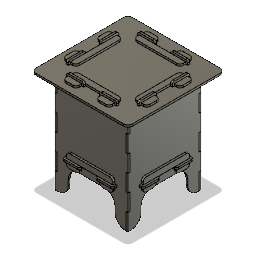
Laterne in 3D parametrisiert (Autodesk Fusion 360 design; units mm, degrees)
Autodesk Fusion 360 part; units mm, degrees
note: some values were not read from the file. Set by a fixed rule: which sketch regions a step uses.
sketch "Skizze1" plane through (0, 0, 0) normal (0, 1, 0) x (1, 0, 0)
  line L0 (52, -52) -> (-52, -52)
  line L1 (-52, -52) -> (-52, 52)
  line L2 (-52, 52) -> (52, 52)
  line L3 (52, 52) -> (52, -52)
  line L4 (52, -52) -> (-52, 52) construction
  line L5 (-52, -52) -> (52, 52) construction
  line L6 (-12, 52) -> (-38, 52)
  line L7 (-38, 52) -> (-38, 58)
  line L8 (-35, 61) -> (-15, 61)
  line L9 (-12, 58) -> (-12, 52)
  line L10 (0, 52) -> (0, -52) construction
  line L11 (-52, 0) -> (52, 0) construction
  line L12 (-35, 55) -> (-15, 55)
  line L13 (-15, 55) -> (-15, 58)
  line L14 (-15, 58) -> (-35, 58)
  line L15 (-35, 58) -> (-35, 55)
  arc A0 (-35, 61) -> (-38, 58) centre (-35, 58) ccw
  arc A1 (-12, 58) -> (-15, 61) centre (-15, 58) ccw
  line L16 (38, 52) -> (38, 58)
  arc A2 (38, 58) -> (35, 61) centre (35, 58) ccw
  line L17 (35, 61) -> (15, 61)
  arc A3 (15, 61) -> (12, 58) centre (15, 58) ccw
  line L18 (12, 58) -> (12, 52)
  line L19 (35, 55) -> (15, 55)
  line L20 (15, 55) -> (15, 58)
  line L21 (15, 58) -> (35, 58)
  line L22 (35, 58) -> (35, 55)
  line L23 (55, 35) -> (55, 15)
  line L24 (55, 15) -> (58, 15)
  line L25 (58, 12) -> (52, 12)
  line L26 (52, 38) -> (58, 38)
  line L27 (61, 35) -> (61, 15)
  arc A4 (61, 35) -> (58, 38) centre (58, 35) ccw
  arc A5 (58, 12) -> (61, 15) centre (58, 15) ccw
  line L28 (58, 35) -> (55, 35)
  line L29 (58, 15) -> (58, 35)
  line L30 (52, -38) -> (58, -38)
  line L31 (61, -35) -> (61, -15)
  line L32 (55, -35) -> (55, -15)
  line L33 (55, -15) -> (58, -15)
  line L34 (58, -15) -> (58, -35)
  arc A6 (61, -15) -> (58, -12) centre (58, -15) ccw
  arc A7 (58, -38) -> (61, -35) centre (58, -35) ccw
  line L35 (58, -35) -> (55, -35)
  line L36 (58, -12) -> (52, -12)
  line L37 (-35, -55) -> (-15, -55)
  line L38 (-35, -61) -> (-15, -61)
  line L39 (-15, -55) -> (-15, -58)
  line L40 (-35, -58) -> (-35, -55)
  arc A8 (-38, -58) -> (-35, -61) centre (-35, -58) ccw
  line L41 (-12, -58) -> (-12, -52)
  line L42 (-38, -52) -> (-38, -58)
  line L43 (35, -61) -> (15, -61)
  line L44 (-15, -58) -> (-35, -58)
  line L45 (12, -58) -> (12, -52)
  line L46 (35, -55) -> (15, -55)
  line L47 (35, -58) -> (35, -55)
  line L48 (15, -55) -> (15, -58)
  arc A9 (-15, -61) -> (-12, -58) centre (-15, -58) ccw
  arc A10 (35, -61) -> (38, -58) centre (35, -58) ccw
  arc A11 (12, -58) -> (15, -61) centre (15, -58) ccw
  line L49 (15, -58) -> (35, -58)
  line L50 (38, -52) -> (38, -58)
  arc A12 (-58, 38) -> (-61, 35) centre (-58, 35) ccw
  line L51 (-55, 15) -> (-58, 15)
  line L52 (-55, -35) -> (-55, -15)
  line L53 (-55, 35) -> (-55, 15)
  line L54 (-58, 35) -> (-55, 35)
  line L55 (-55, -15) -> (-58, -15)
  line L56 (-58, -35) -> (-55, -35)
  line L57 (-58, -15) -> (-58, -35)
  arc A13 (-61, 15) -> (-58, 12) centre (-58, 15) ccw
  line L58 (-58, 12) -> (-52, 12)
  line L59 (-58, 15) -> (-58, 35)
  arc A14 (-61, -35) -> (-58, -38) centre (-58, -35) ccw
  line L60 (-61, -35) -> (-61, -15)
  line L61 (-52, 38) -> (-58, 38)
  line L62 (-58, -12) -> (-52, -12)
  arc A15 (-58, -12) -> (-61, -15) centre (-58, -15) ccw
  line L63 (-61, 35) -> (-61, 15)
  line L64 (-52, -38) -> (-58, -38)
  point P0 (-38, 61)
  point P1 (-12, 61)
  point P2 (61, -38)
  point P3 (61, -12)
  point P4 (12, -61)
  point P5 (38, -61)
  point P6 (-52, -52)
  point P7 (-61, 38)
  point P8 (-52, 0)
  point P9 (-61, 12)
  dimension "d5" = 104
  dimension "d6" = 104
  dimension "d8" = 9
  dimension "d9" = 26
  dimension "d12" = 3
  dimension "d13" = 20
  dimension "d14" = 3
  dimension "d15" = 3
  dimension "d16" = 3
  dimension "d28" = 15
  measures "d5" distance of L1.end L2.end
  measures "d6" distance of P6 L1.end
  measures "d8" distance of L6.start P1
  measures "d9" distance of P0 P1
  measures "d12" distance of L7 L15
  measures "d13" distance of L12.start L12.end
  measures "d14" distance of L6 L12
  measures "d15" distance of L12.end L13.end
  measures "d16" radius of A0
  measures "d28" distance of L10 L13
extrude "Extrusion1" add sketch "Skizze1" along normal blind 3 makes body 1 in component "Boden"
sketch "Skizze2" plane through (-52, 0, 0) normal (-1, 0, 0) x (0, 0, 1)
  line L0 (-12, 0) -> (12, 0) construction
  line L1 (12, 0) -> (12, 3) construction
  line L2 (12, 3) -> (-12, 3)
  line L3 (-12, 3) -> (-12, 0)
  line L4 (-55, 3) -> (55, 3) construction
  line L5 (55, 3) -> (55, 103)
  line L6 (55, 103) -> (-55, 103)
  line L7 (-55, 103) -> (-55, 3)
  line L8 (-55, 3) -> (55, 103) construction
  line L9 (55, 3) -> (-55, 103) construction
  line L10 (-58, 3) -> (-52, 3)
  line L11 (0, 53) -> (0, 3) construction
  line L12 (0, 3) -> (0, 0) construction
  line L13 (-55, 3) -> (55, 3) construction
  line L14 (55, 3) -> (55, 0) construction
  line L15 (-55, 0) -> (-55, 3)
  line L16 (-38, 103) -> (-12, 103)
  line L17 (-12, 103) -> (-12, 109)
  line L18 (-15, 112) -> (-35, 112)
  line L19 (-38, 109) -> (-38, 103)
  line L20 (0, 53) -> (0, 103) construction
  line L21 (-35, 109) -> (-15, 109)
  line L22 (-15, 109) -> (-15, 106)
  line L23 (-15, 106) -> (-35, 106)
  line L24 (-35, 106) -> (-35, 109)
  arc A0 (-35, 112) -> (-38, 109) centre (-35, 109) ccw
  arc A1 (-12, 109) -> (-15, 112) centre (-15, 109) ccw
  line L25 (15, 112) -> (35, 112)
  line L26 (35, 106) -> (35, 109)
  line L27 (38, 109) -> (38, 103)
  line L28 (15, 106) -> (35, 106)
  line L29 (15, 109) -> (15, 106)
  arc A2 (38, 109) -> (35, 112) centre (35, 109) ccw
  line L30 (12, 103) -> (12, 109)
  arc A3 (15, 112) -> (12, 109) centre (15, 109) ccw
  line L31 (35, 109) -> (15, 109)
  line L32 (-35, -26) -> (-35, -34)
  line L33 (-51, -50) -> (-55, -50)
  line L34 (-55, -50) -> (-55, 0)
  line L35 (35, -26) -> (35, -34)
  line L36 (51, -50) -> (55, -50)
  line L37 (55, -50) -> (55, 0)
  line L38 (19, -10) -> (-19, -10)
  arc A4 (-51, -50) -> (-35, -34) centre (-51, -34) ccw
  arc A5 (35, -34) -> (51, -50) centre (51, -34) ccw
  arc A6 (-19, -10) -> (-35, -26) centre (-19, -26) ccw
  arc A7 (35, -26) -> (19, -10) centre (19, -26) ccw
  line L39 (55, 103) -> (52, 103)
  line L40 (52, 103) -> (52, -50)
  line L41 (52, -50) -> (55, -50)
  line L42 (55, -50) -> (55, 103)
  line L43 (-55, 103) -> (-52, 103)
  line L44 (-52, 103) -> (-52, -50)
  line L45 (-52, -50) -> (-55, -50)
  line L46 (-55, -50) -> (-55, 103)
  line L47 (-55, 0) -> (55, 0) construction
  line L48 (55, 77.5) -> (52, 77.5)
  line L49 (55, 52) -> (52, 52)
  line L50 (55, 26.5) -> (52, 26.5)
  line L51 (55, 1) -> (52, 1)
  line L52 (55, -24.5) -> (52, -24.5)
  line L53 (-55, 77.5) -> (-52, 77.5)
  line L54 (-55, 52) -> (-52, 52)
  line L55 (-55, 26.5) -> (-52, 26.5)
  line L56 (-55, 1) -> (-52, 1)
  line L57 (-55, -24.5) -> (-52, -24.5)
  point P0 (0, 53)
  point P1 (55, 0)
  point P2 (-35, -50)
  point P3 (35, -50)
  dimension "d19" = 110
  dimension "d21" = 100
  dimension "d29" = 9
  dimension "d30" = 20
  dimension "d31" = 3
  dimension "d32" = 3
  dimension "d33" = 3
  dimension "d34" = 3
  dimension "d35" = 15
  dimension "d36" = 3
  dimension "d43" = 20
  dimension "d44" = 20
  dimension "d47" = 16
  dimension "d49" = 16
  dimension "d51" = 3
  dimension "d52" = 3
  dimension "d66" = 50
  dimension "d67" = 3
  dimension "d68" = 25.5
  dimension "d71" = -25.5
  dimension "d72" = 0
  dimension "d73" = 40
  dimension "d74" = 3
  measures "d19" distance of L5.end L6.end
  measures "d21" distance of L4.end L5.end
  measures "d29" distance of L16 L18
  measures "d30" distance of L22 L24
  measures "d31" distance of L19 L24
  measures "d32" distance of L17 L22
  measures "d33" distance of L16 L23
  measures "d34" distance of L21 L23
  measures "d35" distance of L20 L22
  measures "d36" radius of A0
  measures "d43" distance of P2 L33.end
  measures "d44" distance of P3 L36.end
  measures "d47" radius of A4
  measures "d49" radius of A6
  measures "d51" distance of L5.end L39.end
  measures "d52" distance of L44 L46
  measures "d66" distance of L36 L47
  measures "d67" distance of L48.start L48.end
  measures "d68" distance of L6 L48
  measures "d73" distance of L36 L38
  measures "d74" distance of L4 L47
extrude "Extrusion1'" add sketch "Skizze2" along normal blind 3 separate body contours L5 L40 L42 L49 L50 | L37 L40 L42 L51 L52 | L6 L16 L32 L33 L35 L36 L38 A4 A5 A6 A7 L40 L44 | L5 L6 L39 L40 L42 L48 | L6 L25 L27 A2 L30 A3 | L6 L16 L17 L18 L19 A0 A1 | L7 L44 L46 L53 L54 | L7 L10 L44 L46 L55 | L33 L34 L44 L45 L46 L57 | L10 L15 L44 L46 L56 makes body 2 in component "Seite"
combine "Kombinieren1" operation cut target body 2 tool bodies 1 keep tools in component "Seite"
other "C-Anordnung2"
sketch "Skizze4" plane through (0, 103, 0) normal (0, 1, 0) x (-1, 0, 0)
  line L0 (55, -52) -> (38, -52)
  line L1 (38, -52) -> (38, -55)
  line L2 (38, -55) -> (55, -55)
  line L3 (55, -55) -> (55, -52)
  line L4 (-66, 73) -> (66, 73)
  line L5 (73, 66) -> (73, -66)
  line L6 (66, -73) -> (-66, -73)
  line L7 (-73, -66) -> (-73, 66)
  line L8 (-73, 73) -> (73, -73) construction
  line L9 (70.898, 70.898) -> (-73, -73) construction
  arc A0 (-73, -66) -> (-66, -73) centre (-66, -66) ccw
  arc A1 (-66, 73) -> (-73, 66) centre (-66, 66) ccw
  arc A2 (73, 66) -> (66, 73) centre (66, 66) ccw
  arc A3 (66, -73) -> (73, -66) centre (66, -66) ccw
  dimension "d79" = 146
  dimension "d80" = 146
  dimension "d83" = 7
  dimension "d86" = 73
  dimension "d87" = 85
  measures "d79" distance of L8.end L9.end
  measures "d80" distance of L8.start L9.end
  measures "d83" radius of A0
  measures "d86" distance of origin L4
extrude "Extrusion1''" add sketch "Skizze4" along normal blind 3 separate body contours L0 L1 L2 L3 | L4 L5 L6 L7 A0 A1 A2 A3 makes body 3 in component "Deckel"
combine "Kombinieren1'" operation cut target body 3 tool bodies 2 keep tools in component "Deckel"
combine "Kombinieren2" operation cut target body 3 tool bodies 2 body 2 seen with x (0, 0, -1) y (0, 1, 0) z (1, 0, 0) at (0, 0, 0) keep tools in component "Deckel"
combine "Kombinieren3" operation cut target body 3 tool bodies 2 body 2 seen with x (-1, 0, 0) y (0, 1, 0) z (0, 0, -1) at (0, 0, 0) keep tools in component "Deckel"
combine "Kombinieren4" operation cut target body 3 tool bodies 2 body 2 seen with x (0, 0, 1) y (0, 1, 0) z (-1, 0, 0) at (0, 0, 0) keep tools in component "Deckel"
sketch "Skizze5" plane through (0, 106, 0) normal (0, 1, 0) x (-1, 0, 0)
  line L0 (-38, -52) -> (-12, -52)
  line L1 (-12, -52) -> (-12, -55)
  line L2 (-12, -55) -> (-38, -55)
  line L3 (-38, -55) -> (-38, -52)
  line L4 (12, -52) -> (38, -52)
  line L5 (38, -52) -> (38, -55)
  line L6 (38, -55) -> (12, -55)
  line L7 (12, -55) -> (12, -52)
  line L8 (-52, 38) -> (-52, 12)
  line L9 (-52, 12) -> (-55, 12)
  line L10 (-55, 12) -> (-55, 38)
  line L11 (-55, 38) -> (-52, 38)
  line L12 (-52, -12) -> (-52, -38)
  line L13 (-52, -38) -> (-55, -38)
  line L14 (-55, -38) -> (-55, -12)
  line L15 (-55, -12) -> (-52, -12)
  line L16 (38, 52) -> (12, 52)
  line L17 (12, 52) -> (12, 55)
  line L18 (12, 55) -> (38, 55)
  line L19 (38, 55) -> (38, 52)
  line L20 (-12, 52) -> (-38, 52)
  line L21 (-38, 52) -> (-38, 55)
  line L22 (-38, 55) -> (-12, 55)
  line L23 (-12, 55) -> (-12, 52)
  line L24 (52, -38) -> (52, -12)
  line L25 (52, -12) -> (55, -12)
  line L26 (55, -12) -> (55, -38)
  line L27 (55, -38) -> (52, -38)
  line L28 (52, 12) -> (52, 38)
  line L29 (52, 38) -> (55, 38)
  line L30 (55, 38) -> (55, 12)
  line L31 (55, 12) -> (52, 12)
  arc A0 (-73, -66) -> (-66, -73) centre (-66, -66) ccw
  line L32 (-66, -73) -> (66, -73)
  arc A1 (66, -73) -> (73, -66) centre (66, -66) ccw
  line L33 (73, -66) -> (73, 66)
  arc A2 (73, 66) -> (66, 73) centre (66, 66) ccw
  line L34 (66, 73) -> (-66, 73)
  arc A3 (-66, 73) -> (-73, 66) centre (-66, 66) ccw
  line L35 (-73, 66) -> (-73, -66)
  line L36 (35, 45) -> (35, 35)
  line L37 (30, 30) -> (-30, 30)
  line L38 (-35, 35) -> (-35, 45)
  line L39 (-30, 50) -> (-20, 50)
  line L40 (-15, 45) -> (-15, 38.5)
  line L41 (-15, 38.5) -> (15, 38.5)
  line L42 (15, 38.5) -> (15, 45)
  line L43 (20, 50) -> (30, 50)
  arc A4 (30, 30) -> (35, 35) centre (30, 35) ccw
  arc A5 (-35, 35) -> (-30, 30) centre (-30, 35) ccw
  arc A6 (-30, 50) -> (-35, 45) centre (-30, 45) ccw
  arc A7 (-15, 45) -> (-20, 50) centre (-20, 45) ccw
  arc A8 (20, 50) -> (15, 45) centre (20, 45) ccw
  arc A9 (35, 45) -> (30, 50) centre (30, 45) ccw
  point P0 (35, 50)
  point P1 (-35, 50)
  point P2 (-15, 50)
  point P3 (15, 50)
  dimension "d88" = 20
  dimension "d89" = 20
  dimension "d90" = 30
  dimension "d92" = 5
  dimension "d94" = 20
  dimension "d95" = 8.5
  measures "d88" distance of P1 P2
  measures "d89" distance of P0 P3
  measures "d90" distance of L40.end L41.end
  measures "d92" radius of A4
  measures "d94" distance of L37 L43
  measures "d95" distance of L37 L41
extrude "Extrusion1'''" add sketch "Skizze5" along normal blind 3 separate body contours L36 L37 L38 L39 L40 L41 L42 L43 A4 A5 A6 A7 A8 A9 makes body 4 in component "Riegel"
other "C-Anordnung3"
other "C-Anordnung4"
sketch "Skizze6" plane through (0, 3, 0) normal (0, 1, 0) x (-1, 0, 0)
  line L0 (15, 55) -> (15, 58)
  line L1 (15, 58) -> (35, 58)
  line L2 (35, 58) -> (35, 55)
  line L3 (35, 55) -> (15, 55)
  line L4 (35, -55) -> (35, -58)
  line L5 (35, -58) -> (15, -58)
  line L6 (15, -58) -> (15, -55)
  line L7 (15, -55) -> (35, -55)
  line L8 (58, 35) -> (58, 15)
  line L9 (58, 15) -> (55, 15)
  line L10 (55, 15) -> (55, 35)
  line L11 (55, 35) -> (58, 35)
  line L12 (-58, 15) -> (-58, 35)
  line L13 (-58, 35) -> (-55, 35)
  line L14 (-55, 35) -> (-55, 15)
  line L15 (-55, 15) -> (-58, 15)
  line L16 (-35, 58) -> (-15, 58)
  line L17 (-15, 58) -> (-15, 55)
  line L18 (-15, 55) -> (-35, 55)
  line L19 (-35, 55) -> (-35, 58)
  line L20 (-58, -35) -> (-58, -15)
  line L21 (-58, -15) -> (-55, -15)
  line L22 (-55, -15) -> (-55, -35)
  line L23 (-55, -35) -> (-58, -35)
  line L24 (55, -15) -> (58, -15)
  line L25 (58, -15) -> (58, -35)
  line L26 (58, -35) -> (55, -35)
  line L27 (55, -35) -> (55, -15)
  line L28 (-15, -58) -> (-35, -58)
  line L29 (-35, -58) -> (-35, -55)
  line L30 (-35, -55) -> (-15, -55)
  line L31 (-15, -55) -> (-15, -58)
  line L32 (38, 52) -> (38, 58)
  arc A0 (38, 58) -> (35, 61) centre (35, 58) ccw
  line L33 (35, 61) -> (15, 61)
  arc A1 (15, 61) -> (12, 58) centre (15, 58) ccw
  line L34 (12, 58) -> (12, 52)
  line L35 (12, 52) -> (-12, 52)
  line L36 (-12, 52) -> (-12, 58)
  arc A2 (-12, 58) -> (-15, 61) centre (-15, 58) ccw
  line L37 (-15, 61) -> (-35, 61)
  arc A3 (-35, 61) -> (-38, 58) centre (-35, 58) ccw
  line L38 (-38, 58) -> (-38, 52)
  line L39 (-38, 52) -> (-52, 52)
  line L40 (-52, 52) -> (-52, 38)
  line L41 (-52, 38) -> (-58, 38)
  arc A4 (-58, 38) -> (-61, 35) centre (-58, 35) ccw
  line L42 (-61, 35) -> (-61, 15)
  arc A5 (-61, 15) -> (-58, 12) centre (-58, 15) ccw
  line L43 (-58, 12) -> (-52, 12)
  line L44 (-52, 12) -> (-52, -12)
  line L45 (-52, -12) -> (-58, -12)
  arc A6 (-58, -12) -> (-61, -15) centre (-58, -15) ccw
  line L46 (-61, -15) -> (-61, -35)
  arc A7 (-61, -35) -> (-58, -38) centre (-58, -35) ccw
  line L47 (-58, -38) -> (-52, -38)
  line L48 (-52, -38) -> (-52, -52)
  line L49 (-52, -52) -> (-38, -52)
  line L50 (-38, -52) -> (-38, -58)
  arc A8 (-38, -58) -> (-35, -61) centre (-35, -58) ccw
  line L51 (-35, -61) -> (-15, -61)
  arc A9 (-15, -61) -> (-12, -58) centre (-15, -58) ccw
  line L52 (-12, -58) -> (-12, -52)
  line L53 (-12, -52) -> (12, -52)
  line L54 (12, -52) -> (12, -58)
  arc A10 (12, -58) -> (15, -61) centre (15, -58) ccw
  line L55 (15, -61) -> (35, -61)
  arc A11 (35, -61) -> (38, -58) centre (35, -58) ccw
  line L56 (38, -58) -> (38, -52)
  line L57 (38, -52) -> (52, -52)
  line L58 (52, -52) -> (52, -38)
  line L59 (52, -38) -> (58, -38)
  arc A12 (58, -38) -> (61, -35) centre (58, -35) ccw
  line L60 (61, -35) -> (61, -15)
  arc A13 (61, -15) -> (58, -12) centre (58, -15) ccw
  line L61 (58, -12) -> (52, -12)
  line L62 (52, -12) -> (52, 12)
  line L63 (52, 12) -> (58, 12)
  arc A14 (58, 12) -> (61, 15) centre (58, 15) ccw
  line L64 (61, 15) -> (61, 35)
  arc A15 (61, 35) -> (58, 38) centre (58, 35) ccw
  line L65 (58, 38) -> (52, 38)
  line L66 (52, 38) -> (52, 52)
  line L67 (52, 52) -> (38, 52)
sketch "Skizze7" plane through (-55, 0, 0) normal (-1, 0, 0) x (0, 0, 1)
  line L0 (12, 0) -> (12, 3)
  line L1 (12, 3) -> (38, 3)
  line L2 (38, 3) -> (38, 0)
  line L3 (38, 0) -> (12, 0)
  line L4 (-38, 0) -> (-38, 3)
  line L5 (-38, 3) -> (-12, 3)
  line L6 (-12, 3) -> (-12, 0)
  line L7 (-12, 0) -> (-38, 0)
  line L8 (-15, 106) -> (-35, 106)
  line L9 (-35, 106) -> (-35, 109)
  line L10 (-35, 109) -> (-15, 109)
  line L11 (-15, 109) -> (-15, 106)
  line L12 (15, 109) -> (35, 109)
  line L13 (35, 109) -> (35, 106)
  line L14 (35, 106) -> (15, 106)
  line L15 (15, 106) -> (15, 109)
  arc A0 (-51, -50) -> (-35, -34) centre (-51, -34) ccw
  line L16 (-35, -34) -> (-35, -26)
  arc A1 (-19, -10) -> (-35, -26) centre (-19, -26) ccw
  line L17 (-19, -10) -> (19, -10)
  arc A2 (35, -26) -> (19, -10) centre (19, -26) ccw
  line L18 (35, -26) -> (35, -34)
  arc A3 (35, -34) -> (51, -50) centre (51, -34) ccw
  line L19 (52, -50) -> (52, -24.5)
  line L20 (52, -24.5) -> (55, -24.5)
  line L21 (55, -24.5) -> (55, 1)
  line L22 (55, 1) -> (52, 1)
  line L23 (52, 1) -> (52, 26.5)
  line L24 (52, 26.5) -> (55, 26.5)
  line L25 (55, 26.5) -> (55, 52)
  line L26 (55, 52) -> (52, 52)
  line L27 (52, 52) -> (52, 77.5)
  line L28 (52, 77.5) -> (55, 77.5)
  line L29 (55, 77.5) -> (55, 103)
  line L30 (55, 103) -> (38, 103)
  line L31 (38, 103) -> (38, 109)
  arc A4 (38, 109) -> (35, 112) centre (35, 109) ccw
  line L32 (35, 112) -> (15, 112)
  arc A5 (15, 112) -> (12, 109) centre (15, 109) ccw
  line L33 (12, 109) -> (12, 103)
  line L34 (12, 103) -> (-12, 103)
  line L35 (-12, 103) -> (-12, 109)
  arc A6 (-12, 109) -> (-15, 112) centre (-15, 109) ccw
  line L36 (-15, 112) -> (-35, 112)
  arc A7 (-35, 112) -> (-38, 109) centre (-35, 109) ccw
  line L37 (-38, 109) -> (-38, 103)
  line L38 (-38, 103) -> (-52, 103)
  line L39 (-52, 103) -> (-52, 77.5)
  line L40 (-52, 77.5) -> (-55, 77.5)
  line L41 (-55, 77.5) -> (-55, 52)
  line L42 (-55, 52) -> (-52, 52)
  line L43 (-52, 52) -> (-52, 26.5)
  line L44 (-52, 26.5) -> (-55, 26.5)
  line L45 (-55, 26.5) -> (-55, 1)
  line L46 (-55, 1) -> (-52, 1)
  line L47 (-52, 1) -> (-52, -24.5)
  line L48 (-52, -24.5) -> (-55, -24.5)
  line L49 (-55, -24.5) -> (-55, -50)
  line L50 (-55, -50) -> (-51, -50)
  line L51 (51, -50) -> (52, -50)
sketch "Skizze8" plane through (0, 106, 0) normal (0, 1, 0) x (-1, 0, 0)
  line L0 (-38, -52) -> (-12, -52)
  line L1 (-12, -52) -> (-12, -55)
  line L2 (-12, -55) -> (-38, -55)
  line L3 (-38, -55) -> (-38, -52)
  line L4 (12, -52) -> (38, -52)
  line L5 (38, -52) -> (38, -55)
  line L6 (38, -55) -> (12, -55)
  line L7 (12, -55) -> (12, -52)
  line L8 (-52, 38) -> (-52, 12)
  line L9 (-52, 12) -> (-55, 12)
  line L10 (-55, 12) -> (-55, 38)
  line L11 (-55, 38) -> (-52, 38)
  line L12 (-52, -12) -> (-52, -38)
  line L13 (-52, -38) -> (-55, -38)
  line L14 (-55, -38) -> (-55, -12)
  line L15 (-55, -12) -> (-52, -12)
  line L16 (38, 52) -> (12, 52)
  line L17 (12, 52) -> (12, 55)
  line L18 (12, 55) -> (38, 55)
  line L19 (38, 55) -> (38, 52)
  line L20 (-12, 52) -> (-38, 52)
  line L21 (-38, 52) -> (-38, 55)
  line L22 (-38, 55) -> (-12, 55)
  line L23 (-12, 55) -> (-12, 52)
  line L24 (52, -38) -> (52, -12)
  line L25 (52, -12) -> (55, -12)
  line L26 (55, -12) -> (55, -38)
  line L27 (55, -38) -> (52, -38)
  line L28 (52, 12) -> (52, 38)
  line L29 (52, 38) -> (55, 38)
  line L30 (55, 38) -> (55, 12)
  line L31 (55, 12) -> (52, 12)
  arc A0 (-73, -66) -> (-66, -73) centre (-66, -66) ccw
  line L32 (-66, -73) -> (66, -73)
  arc A1 (66, -73) -> (73, -66) centre (66, -66) ccw
  line L33 (73, -66) -> (73, 66)
  arc A2 (73, 66) -> (66, 73) centre (66, 66) ccw
  line L34 (66, 73) -> (-66, 73)
  arc A3 (-66, 73) -> (-73, 66) centre (-66, 66) ccw
  line L35 (-73, 66) -> (-73, -66)
sketch "Skizze9" plane through (0, 109, -5) normal (0, 1, 0) x (-1, 0, 0)
  arc A0 (30, 48.5) -> (35, 53.5) centre (30, 53.5) ccw
  line L0 (35, 53.5) -> (35, 63.5)
  arc A1 (35, 63.5) -> (30, 68.5) centre (30, 63.5) ccw
  line L1 (30, 68.5) -> (20, 68.5)
  arc A2 (20, 68.5) -> (15, 63.5) centre (20, 63.5) ccw
  line L2 (15, 63.5) -> (15, 57)
  line L3 (15, 57) -> (-15, 57)
  line L4 (-15, 57) -> (-15, 63.5)
  arc A3 (-15, 63.5) -> (-20, 68.5) centre (-20, 63.5) ccw
  line L5 (-20, 68.5) -> (-30, 68.5)
  arc A4 (-30, 68.5) -> (-35, 63.5) centre (-30, 63.5) ccw
  line L6 (-35, 63.5) -> (-35, 53.5)
  arc A5 (-35, 53.5) -> (-30, 48.5) centre (-30, 53.5) ccw
  line L7 (-30, 48.5) -> (30, 48.5)
component "Boden" placed x (1, 0, 0) y (0, 1, 0) z (0, 0, 1) at (0, 0, 0)
component "Seite" placed x (1, 0, 0) y (0, 1, 0) z (0, 0, 1) at (0, 0, 0)
component "Seite" placed x (0, 0, -1) y (0, 1, 0) z (1, 0, 0) at (0, 0, 0)
component "Seite" placed x (-1, 0, 0) y (0, 1, 0) z (0, 0, -1) at (0, 0, 0)
component "Seite" placed x (0, 0, 1) y (0, 1, 0) z (-1, 0, 0) at (0, 0, 0)
component "Deckel" placed x (1, 0, 0) y (0, 1, 0) z (0, 0, 1) at (0, 0, 0)
component "Riegel" placed x (1, 0, 0) y (0, 1, 0) z (0, 0, 1) at (0, 0, 13.5)
component "Riegel" placed x (0, 0, -1) y (0, 1, 0) z (1, 0, 0) at (13.5, 0, 0)
component "Riegel" placed x (-1, 0, 0) y (0, 1, 0) z (0, 0, -1) at (0, 0, -13.5)
component "Riegel" placed x (0, 0, 1) y (0, 1, 0) z (-1, 0, 0) at (-13.5, 0, 0)
component "Riegel" placed x (1, 0, 0) y (0, 0, 1) z (0, -1, 0) at (0, 41.5, -51)
component "Riegel" placed x (0, 0, -1) y (1, 0, 0) z (0, -1, 0) at (-51, 41.5, 0)
component "Riegel" placed x (-1, 0, 0) y (0, 0, -1) z (0, -1, 0) at (0, 41.5, 51)
component "Riegel" placed x (0, 0, 1) y (-1, 0, 0) z (0, -1, 0) at (51, 41.5, 0)
equation "MaterialDicke = 3 mm"
equation "Oberteil_Hoehe = 100 mm"
equation "Unterteil_Hoehe = 50 mm"
equation "Koerper_Breite = 110 mm"
equation "d5 = Koerper_Breite - 2 * MaterialDicke"
equation "d6 = d5"
equation "Riegel_Breite = 20 mm"
equation "d8 = 3 * MaterialDicke"
equation "d9 = Riegel_Breite + 2 * MaterialDicke"
equation "Riegel_Abstand = 30 mm"
equation "d12 = MaterialDicke"
equation "d13 = Riegel_Breite"
equation "d14 = d12"
equation "d15 = MaterialDicke"
equation "d16 = MaterialDicke"
equation "d17 = MaterialDicke"
equation "d19 = Koerper_Breite"
equation "d21 = Oberteil_Hoehe"
equation "Beine_Laenge = 30 mm"
equation "Beine_Breite = 20 mm"
equation "d28 = Riegel_Abstand / 2"
equation "d29 = MaterialDicke * 3"
equation "d30 = Riegel_Breite"
equation "d31 = MaterialDicke"
equation "d32 = MaterialDicke"
equation "d33 = MaterialDicke"
equation "d34 = MaterialDicke"
equation "d35 = Riegel_Abstand / 2"
equation "d36 = MaterialDicke"
equation "d43 = Beine_Breite"
equation "d44 = Beine_Breite"
equation "d47 = Beine_Radius"
equation "Beine_Radius = 16 mm"
equation "d49 = Beine_Radius"
equation "Gesammthoehe = Oberteil_Hoehe + Unterteil_Hoehe + MaterialDicke"
equation "d51 = MaterialDicke"
equation "d52 = MaterialDicke"
equation "d66 = Unterteil_Hoehe"
equation "d67 = MaterialDicke"
equation "d68 = Gesammthoehe / 6"
equation "d71 = -( Gesammthoehe / 6 )"
equation "d74 = MaterialDicke"
equation "d75 = MaterialDicke"
equation "d79 = d80"
equation "d80 = Koerper_Breite + 2 * Deckel_Ueberhang"
equation "Deckel_Ueberhang = 18 mm"
equation "Deckel_Radius = 7 mm"
equation "d83 = Deckel_Radius"
equation "d84 = MaterialDicke"
equation "d86 = ( Koerper_Breite + 2 * Deckel_Ueberhang ) / 2"
equation "d88 = Riegel_Breite"
equation "d89 = Riegel_Breite"
equation "d90 = Riegel_Abstand"
equation "Riegel_Radius = 5 mm"
equation "Riegel_Hoehe = 20 mm"
equation "d94 = Riegel_Hoehe"
equation "d95 = ( Riegel_Hoehe - MaterialDicke ) / 2"
equation "d96 = MaterialDicke"
